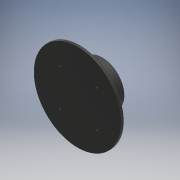
# Autodesk Inventor part: 底座
Saved by Autodesk Inventor 2017 (Build 210142000, 142)
## iProperties
Part Number: 底座
Material: 熱塑性塑膠樹脂
Document SubType Name: Modeling
Designer: Brian
Density: 1.28 g/cm^3
Appearance: 平滑 - 黑色
Mass: 196.131 g
Surface Area: 675.148 cm^2
Volume: 153.227 cm^3
Author: Brian
Autodesk Inventor part; units mm, degrees
ref_plane "YZ Plane" through (0, 0, 0) normal (1, 0, 0) x (0, 1, 0)
ref_plane "XZ Plane" through (0, 0, 0) normal (0, 1, 0) x (-1, 0, 0)
ref_plane "XY Plane" through (0, 0, 0) normal (0, 0, 1) x (1, 0, 0)
sketch "草圖1" plane through (0, 0, 0) normal (0, 1, 0) x (-1, 0, 0)
  circle A0 centre (0, 0) radius 50
  dimension "d0" = 100
  constraints: 1 centre point, 1 coincident
  measures "d0" diameter of A0
extrude "擠出1" add sketch "草圖1" along normal blind 51.6
shell "薄殼1" thickness 3 removed faces 1 at (-9.39, 51.6, -8.8667)
sketch "草圖2" plane through (0, 0, 0) normal (0, -1, 0) x (1, 0, 0)
  circle A0 centre (0, 0) radius 100
  dimension "d4" = 200
  constraints: 1 centre point, 1 coincident
  measures "d4" diameter of A0
extrude "擠出2" add sketch "草圖2" along normal blind 5
sketch "草圖3" plane through (0, 0, 0) normal (0, 1, 0) x (1, 0, 0)
  circle A0 centre (0, 0) radius 60
  line L0 (42.4264, -42.4264) -> (-42.4264, -42.4264)
  line L1 (-42.4264, -42.4264) -> (-42.4264, 42.4264)
  line L2 (-42.4264, 42.4264) -> (42.4264, 42.4264)
  line L3 (42.4264, 42.4264) -> (42.4264, -42.4264)
  line L4 (42.4264, -42.4264) -> (-42.4264, 42.4264) construction
  line L5 (-42.4264, -42.4264) -> (42.4264, 42.4264) construction
  dimension "d7" = 120
  constraints: 12 end point, 2 midpoint, 2 parallel, 2 perpendicular, 1 coincident, 1 horizontal, 3 other
hole "孔1" at (-42.4264, 0, 42.4264) at (-42.4264, 0, -42.4264) at (42.4264, 0, -42.4264) at (42.4264, 0, 42.4264) direction (0, -1, 0) diameter 8 depth 8 tip angle 118
sketch "草圖4" plane through (0, 3, 0) normal (0, 1, 0) x (1, 0, 0)
  line L0 (-10, -20) -> (10, -20)
  line L1 (10, -20) -> (10, -10)
  line L2 (10, -10) -> (-10, -10)
  line L3 (-10, -10) -> (-10, -20)
  line L4 (-10, 30) -> (10, 30)
  line L5 (10, 30) -> (10, 40)
  line L6 (10, 40) -> (-10, 40)
  line L7 (-10, 40) -> (-10, 30)
  point P0 (0, 0)
  dimension "d15" = 10
  dimension "d16" = 30
  dimension "d17" = 10
  dimension "d18" = 10
  dimension "d19" = 20
  dimension "d20" = 10
  constraints: 16 end point, 4 parallel, 2 horizontal, 2 perpendicular, 2 point on line
  measures "d15" distance from line of point (0, 0) L2
  measures "d16" distance from line of point (0, 0) L4
  measures "d17" distance of L6.end L4.start
  measures "d18" distance of L2.end L0.start
  measures "d19" distance of L1.end L2.end
  measures "d20" distance from line of point (0, 0) L7
extrude "擠出3" add sketch "草圖4" along normal blind 30
sketch "草圖5" plane through (0, 33, 0) normal (0, 1, 0) x (1, 0, 0)
  line L0 (5, 34.3) -> (-5, 34.3)
  line L1 (-5, 34.3) -> (-5, -14.3)
  line L2 (-5, -14.3) -> (5, -14.3)
  line L3 (5, -14.3) -> (5, 34.3)
  line L4 (5, 34.3) -> (-5, -14.3) construction
  line L5 (-5, 34.3) -> (5, -14.3) construction
  line L6 (10, 30) -> (10, 40) projected
  line L7 (10, 40) -> (-10, 40) projected
  line L8 (-10, 30) -> (10, 30) projected
  line L9 (16.2048, 30) -> (16.2048, -10)
  line L10 (0, 10) -> (16.2048, 10)
  line L11 (10, -10) -> (-10, -10) projected
  dimension "d23" = 10
  dimension "d24" = 48.6
  dimension "d37" = 5
  constraints: 16 end point, 3 midpoint, 2 horizontal, 2 parallel, 2 point on line, 1 perpendicular, 1 vertical
  measures "d23" distance of L1.end L2.end
  measures "d24" distance of L0.end L1.end
  measures "d37" distance between parallel lines of L6 L3
hole "孔2" at (-5, 33, 14.3) at (5, 33, 14.3) at (5, 33, -34.3) at (-5, 33, -34.3) direction (0, -1, 0) diameter 3 depth 8 tip angle 118
sketch "草圖6" plane through (10, 3, 10) normal (0, 0, -1) x (-1, 0, 0)
  line L0 (20, 0) -> (0, 0) projected
  line L1 (5, 0) -> (15, 0)
  line L2 (15, 0) -> (15, 20)
  line L3 (15, 20) -> (5, 20)
  line L4 (5, 20) -> (5, 0)
  line L5 (0, 0) -> (0, 30) projected
  line L6 (20, 0) -> (20, 30) projected
  point P0 (10, -3)
  dimension "d32" = 5
  dimension "d33" = 5
  dimension "d34" = 20
  constraints: 8 end point, 2 parallel, 1 horizontal, 1 perpendicular, 1 point on line
  measures "d32" distance between parallel lines of L5 L4
  measures "d33" distance between parallel lines of L6 L2
  measures "d34" distance of L1.end L2.end
extrude "擠出4" cut sketch "草圖6" against normal through all
fillet "圓角1" radius 5 2 edges at (5, 23, 15) (-5, 23, 15)
